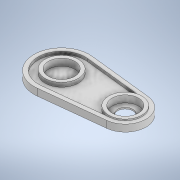
# Autodesk Inventor part: Abdeckung
Saved by Autodesk Inventor 2021 (Build 250183000, 183)
## iProperties
Created: 2021-01-19
Part Number: Abdeckung
Material: Generisch
Document SubType Name: Modeling
Designer: Jaro Machnow
Density: 1 g/cm^3
Appearance: Vorgabe
Author: Jaro Machnow
Autodesk Inventor part; units mm, degrees
ref_plane "YZ Plane" through (0, 0, 0) normal (1, 0, 0) x (0, 1, 0)
ref_plane "XZ Plane" through (0, 0, 0) normal (0, 1, 0) x (-1, 0, 0)
ref_plane "XY Plane" through (0, 0, 0) normal (0, 0, 1) x (1, 0, 0)
sketch "Skizze1" plane through (0, 0, 0) normal (0, 1, 0) x (-1, 0, 0)
  arc A0 (-2.173913, -19.881502) -> (-2.173913, 19.881502) centre (0, 0) ccw
  arc A1 (-47.630435, 14.911126) -> (-47.630435, -14.911126) centre (-46, 0) ccw
  line L0 (-2.173913, 19.881502) -> (-47.630435, 14.911126)
  line L1 (-2.173913, -19.881502) -> (-47.630435, -14.911126)
  line L2 (45.02348, 0) -> (-115.148005, 0) construction
  dimension "d0" = 40
  dimension "d1" = 30
  dimension "d2" = 46
  constraints: 6 end point, 4 point on circle, 4 tangent, 2 centre point, 2 horizontal, 1 coincident, 1 point on line
  measures "d0" diameter of A0
  measures "d1" diameter of A1
  measures "d2" distance of A1.centre point (0, 0)
extrude "Extrusion1" add sketch "Skizze1" along normal blind 5
shell "Wandung1" thickness 3 removed faces 1 at (17.326087, 5, -4.970375)
sketch "Skizze2" plane through (0, 3, 0) normal (0, 1, 0) x (1, 0, 0)
  circle A0 centre (0, 0) radius 9.5
  circle A1 centre (0, 0) radius 12
  dimension "d6" = 19
  dimension "d7" = 24
  constraints: 2 centre point, 2 coincident
  measures "d6" diameter of A0
  measures "d7" diameter of A1
extrude "Extrusion2" add sketch "Skizze2" along normal blind 3
sketch "Skizze3" plane through (0, 3, 0) normal (0, 1, 0) x (1, 0, 0)
  arc A0 (47.304348, -11.928901) -> (47.304348, 11.928901) centre (46, 0) ccw
  circle A1 centre (46, 0) radius 9.5
  circle A2 centre (46, 0) radius 12
  point P0 (0, 0)
  point P1 (47.304348, -11.928901)
  dimension "d10" = 19
  constraints: 2 centre point, 2 coincident
  measures "d10" diameter of A1
extrude "Extrusion3" add sketch "Skizze3" along normal blind 3
sketch "Skizze4" plane through (0, 3, 0) normal (0, 1, 0) x (1, 0, 0)
  circle A0 centre (0, 0) radius 9.5
  constraints: 1 centre point, 1 coincident
extrude "Extrusion4" cut sketch "Skizze4" against normal blind 2
sketch "Skizze5" plane through (46, 3, 0) normal (0, 1, 0) x (1, 0, 0)
  circle A0 centre (0, 0) radius 9.5
  point P0 (-46, 0)
  constraints: 1 centre point
extrude "Extrusion5" cut sketch "Skizze5" against normal blind 2
sketch "Skizze6" plane through (46, 1, 0) normal (0, 1, 0) x (1, 0, 0)
  point P0 (-46, 0)
  point P1 (0, 0)
  point P2 (0, 0)
  constraints: 1 coincident
hole "Bohrung1" at (46, 1, 0) direction (0, -1, 0) diameter 11 end through all
